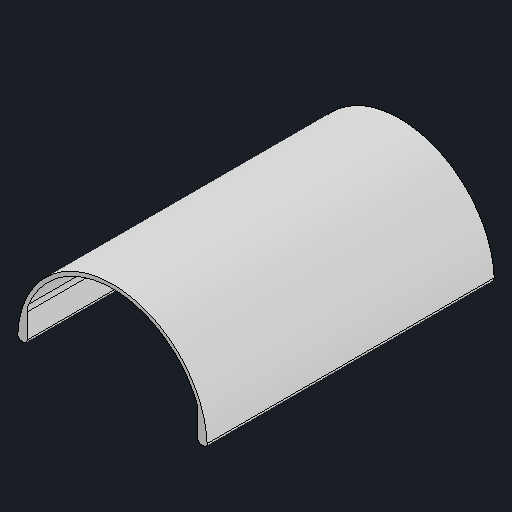
# Autodesk Inventor part: Parts-Tray-for-plasma-vessel
Saved by Autodesk Inventor 2025 (Build 290162000, 162)
## iProperties
Created: 2024-06-21
Part Number: Parts-Tray-for-plasma-vessel
Material: Generic
Document SubType Name: Modeling
Designer: queezz
Density: 1 g/cm^3
Appearance: Default
Author: queezz
Autodesk Inventor part; units mm, degrees
ref_plane "YZ Plane" through (0, 0, 0) normal (1, 0, 0) x (0, 1, 0)
ref_plane "XZ Plane" through (0, 0, 0) normal (0, 1, 0) x (-1, 0, 0)
ref_plane "XY Plane" through (0, 0, 0) normal (0, 0, 1) x (1, 0, 0)
sketch "Sketch1" plane through (0, 0, 0) normal (0, 0, 1) x (1, 0, 0)
  arc A0 (49.5, 0) -> (-49.5, 0) centre (0, 0) ccw
  arc A1 (47.5, 0) -> (-47.5, 0) centre (0, 0) ccw
  line L0 (47.5, 0) -> (49.5, 0)
  line L1 (-47.5, 0) -> (-49.5, 0)
  line L2 (-49.5, 0) -> (-44.5, 0)
  line L3 (-44.5, 0) -> (-44.5, 16.6132)
  line L4 (49.5, 0) -> (44.5, 0)
  line L5 (44.5, 0) -> (44.5, 16.6132)
  point P0 (-47.5, 0)
  dimension "d0" = 99
  dimension "d1" = 2
  dimension "d4" = 5
  dimension "d6" = 5
  constraints: 12 end point, 6 point on circle, 3 horizontal, 2 centre point, 2 coincident, 2 horizontal alignment, 1 perpendicular, 1 point on line, 1 vertical
  measures "d0" diameter of A0
  measures "d1" radial gap between concentric circles of A0 A1
  measures "d4" distance from line of L1.end L3
  measures "d6" distance of L0.end L4.end
extrude "Extrusion1" add sketch "Sketch1" along normal blind 150
fillet "Fillet1" radius 2 4 edges at (-44.5, 0, 75) (-49.5, 0, 75) (44.5, 0, 75) (49.5, 0, 75)
fillet "Fillet2" radius 10 2 edges at (-44.5, 16.6132, 75) (44.5, 16.6132, 75)
equation "\"d1\" = 2 * extrusion_width"
equation "\"extrusion_width\" = 1"
body "Solid1"
